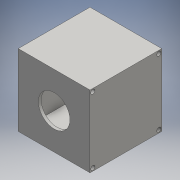
# Autodesk Inventor part: 50x50Motor
Saved by Autodesk Inventor 2016 (Build 200138000, 138)
## iProperties
Created: 2016-05-22
Part Number: 50x50Motor
Material: Generic
Document SubType Name: Modeling
Designer: Kurtis
Density: 1 g/cm^3
Appearance: Default
Author: Kurtis
Autodesk Inventor part; units mm, degrees
ref_plane "YZ Plane" through (0, 0, 0) normal (1, 0, 0) x (0, 1, 0)
ref_plane "XZ Plane" through (0, 0, 0) normal (0, 1, 0) x (-1, 0, 0)
ref_plane "XY Plane" through (0, 0, 0) normal (0, 0, 1) x (1, 0, 0)
sketch "Sketch1" plane through (0, 0, 0) normal (0, 0, 1) x (1, 0, 0)
  line L0 (-25, -25) -> (25, -25)
  line L1 (25, -25) -> (25, 25)
  line L2 (25, 25) -> (-25, 25)
  line L3 (-25, 25) -> (-25, -25)
  line L4 (-25, -25) -> (25, 25) construction
  line L5 (25, -25) -> (-25, 25) construction
  point P0 (0, 0)
  dimension "d0" = 50
  dimension "d1" = 50
  constraints: 12 end point, 2 midpoint, 2 parallel, 1 horizontal, 1 perpendicular
  measures "d0" distance of L2.end L1.end
  measures "d1" distance of L1.end L0.end
extrude "Main Block" add sketch "Sketch1" along normal blind 50
sketch "Sketch2" plane through (-25, 25, 0) normal (0, 1, 0) x (1, 0, 0)
  line L0 (0, -50) -> (50, -50) construction
  line L1 (0, 0) -> (50, 0) construction
  line L2 (50, -50) -> (0, 0) construction
  line L3 (46, -46) -> (4, -46)
  line L4 (4, -46) -> (4, -4)
  line L5 (4, -4) -> (46, -4)
  line L6 (46, -4) -> (46, -46)
  line L7 (46, -46) -> (4, -4) construction
  line L8 (4, -46) -> (46, -4) construction
  line L9 (25, -25) -> (25, -46) construction
  point P0 (25, 0)
  dimension "d4" = 42
  dimension "d5" = 42
  constraints: 16 end point, 4 midpoint, 2 parallel, 1 horizontal, 1 perpendicular
  measures "d4" distance of L4.end L5.end
  measures "d5" distance of L3.end L4.end
extrude "Motor Void" cut sketch "Sketch2" against normal blind 48
sketch "Sketch3" plane through (-25, 25, 0) normal (0, 1, 0) x (1, 0, 0)
  line L0 (25, 0) -> (25, -4) construction
  line L1 (4, -4) -> (46, -4) construction
  line L2 (16.75, -4) -> (33.25, -4)
  line L3 (33.25, -4) -> (33.25, 0)
  line L4 (33.25, 0) -> (16.75, 0)
  line L5 (16.75, 0) -> (16.75, -4)
  line L6 (16.75, -4) -> (33.25, 0) construction
  line L7 (33.25, -4) -> (16.75, 0) construction
  point P0 (25, -2)
  dimension "d8" = 16.5
  dimension "d9" = 4
  constraints: 14 end point, 4 midpoint, 2 parallel, 1 horizontal, 1 perpendicular
  measures "d8" distance of L4.end L3.end
  measures "d9" distance of L3.end L2.end
extrude "Cable Void" cut sketch "Sketch3" against normal blind 21
sketch "Sketch4" plane through (-25, -25, 0) normal (0, -1, 0) x (1, 0, 0)
  line L0 (0, 0) -> (0, 50) construction
  line L1 (50, 50) -> (0, 50) construction
  line L2 (0, 0) -> (50, 50) construction
  circle A0 centre (25, 25) radius 11
  point P0 (25, 0)
  dimension "d12" = 22
  constraints: 2 end point, 1 centre point, 1 midpoint
  measures "d12" diameter of A0
extrude "Raised Void" cut sketch "Sketch4" against normal blind 2
sketch "Sketch5" plane through (-25, -25, 0) normal (-1, 0, 0) x (0, 0, 1)
  line L0 (0, 0) -> (0, 50) construction
  line L1 (4, 50) -> (4, 2) construction
  line L2 (0, 50) -> (4, 50) construction
  line L3 (0, 50) -> (50, 50) construction
  line L4 (46, 2) -> (4, 2) construction
  line L5 (4, 50) -> (4, 2) construction
  line L6 (4, 2) -> (46, 2) construction
  line L7 (46, 50) -> (46, 2) construction
  line L8 (46, 2) -> (46, 50) construction
  line L9 (50, 0) -> (50, 50) construction
  line L10 (46, 50) -> (50, 50) construction
  line L11 (50, 50) -> (48, 50) construction
  line L12 (48, 50) -> (48, 48) construction
  circle A0 centre (48, 48) radius 1.5
  line L13 (48, 0) -> (48, 2) construction
  line L14 (48, 0) -> (50, 0) construction
  line L15 (0, 50) -> (4, 50) construction
  line L16 (2, 50) -> (2, 48) construction
  line L17 (0, 0) -> (50, 0) construction
  line L18 (2, 0) -> (2, 2) construction
  line L19 (2, 0) -> (4, 0) construction
  circle A1 centre (2, 48) radius 1.5
  circle A2 centre (2, 2) radius 1.5
  circle A3 centre (48, 2) radius 1.5
  point P0 (0, 25)
  dimension "d15" = 2
  dimension "d16" = 3
  dimension "d17" = 2
  dimension "d18" = 90
  dimension "d19" = 2
  dimension "d20" = 2
  dimension "d21" = 90
  dimension "d22" = 3
  dimension "d23" = 3
  dimension "d24" = 3
  dimension "d25" = 2
  dimension "d26" = 48
  dimension "d27" = 2
  constraints: 26 end point, 5 collinear, 5 perpendicular, 4 centre point, 4 coincident, 2 horizontal, 2 midpoint, 2 vertical, 1 point on line
  measures "d15" distance of L11.end L12.end
  measures "d16" diameter of A0
  measures "d17" distance of L13.start L13.end
  measures "d18" angle of L14 L13
  measures "d19" distance of L16.start L16.end
  measures "d20" distance of L18.start L18.end
  measures "d21" angle of L19 L18
  measures "d22" diameter of A1
  measures "d23" diameter of A2
  measures "d24" diameter of A3
  measures "d25" distance between parallel lines of L9 L13
  measures "d26" distance between parallel lines of L9 L18
  measures "d27" distance between parallel lines of L4 L14
extrude "Extrusion5" cut sketch "Sketch5" against normal blind 50
body "Solid1"
